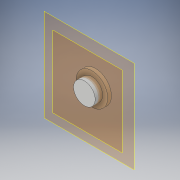
# Autodesk Inventor part: button
Saved by Autodesk Inventor 2019 (Build 230136000, 136)
## iProperties
Created: 2019-08-20
Part Number: button
Material: Generic
Document SubType Name: Modeling
Designer: assman
Density: 1 g/cm^3
Appearance: Default
Author: assman
## iProperties of the stored document button_3DPrint.ipt
Created: 2019-08-20
Part Number: button_3DPrint
Material: Generic
Document SubType Name: Modeling
Designer: assman
Density: 1 g/cm^3
Appearance: Default
Author: assman
Autodesk Inventor part; units mm, degrees
ref_plane "YZ Plane" through (0, 0, 0) normal (1, 0, 0) x (0, 1, 0)
ref_plane "XZ Plane" through (0, 0, 0) normal (0, 1, 0) x (-1, 0, 0)
ref_plane "XY Plane" through (0, 0, 0) normal (0, 0, 1) x (1, 0, 0)
ref_plane "Work Plane1" through (0, 0, 0) normal (0, 0, 1) x (1, 0, 0)
sketch "Sketch1" plane through (0, 0, 0) normal (0, 0, 1) x (1, 0, 0)
  circle A0 centre (0, 0) radius 2.45
  constraints: 1 centre point
extrude "Extrusion1" add sketch "Sketch1" along normal blind 1
sketch "Sketch3" plane through (0, 0, 0) normal (0, 0, -1) x (-1, 0, 0)
  circle A0 centre (0, 0) radius 2.45 projected
  circle A1 centre (0, 0) radius 2.05
  dimension "d4" = 0.4
  constraints: 1 centre point
  measures "d4" radial gap between concentric circles of A0 A1
extrude "Extrusion2" add sketch "Sketch3" along normal blind 2.6
sketch "Sketch4" plane through (0, 0, -2.6) normal (0, 0, -1) x (-1, 0, 0)
  circle A0 centre (0, 0) radius 2.05 projected
  circle A1 centre (0, 0) radius 4.05
  dimension "d7" = 2
  constraints: 1 centre point
  measures "d7" radial gap between concentric circles of A0 A1
extrude "Extrusion3" add sketch "Sketch4" against normal blind 1.2
ref_plane "Work Plane2" through (0, 0, -0.5) normal (0, 0, 1) x (-1, 0, 0)
ref_plane "Work Plane3" through (-4.455, -4.455, -1.2) normal (0, 0, 1) x (1, 0, 0)
thicken "Thicken1" operation add thickness 1 both sides no extend neighbours yes toward (-0.9967573, -0.0804666, 0) faces at (-4.0369, -0.3259, -1.8)
thicken "Thicken2" operation add thickness 1 both sides no extend neighbours yes toward (-0.9870503, 0.1604113, 0) faces at (-2.4183, 0.393, -0.9333) (2.4183, 0.393, 0.6667)
body "Solid1"
